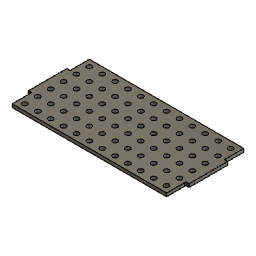
Shelf_Cut1 (Autodesk Fusion 360 design; units mm, degrees)
Autodesk Fusion 360 part; units mm, degrees
sketch "Sketch1" plane through (0, 0, 0) normal (0, 1, 0) x (1, 0, 0)
  line L0 (0, 0) -> (609.6, 0)
  line L1 (609.6, 0) -> (609.6, -304.8)
  line L2 (609.6, -304.8) -> (0, -304.8)
  line L3 (0, -304.8) -> (0, 0)
  line L4 (12.7, -228.6) -> (-12.7, -228.6)
  line L5 (-12.7, -228.6) -> (-12.7, -76.2)
  line L6 (-12.7, -76.2) -> (12.7, -76.2)
  line L7 (12.7, -76.2) -> (12.7, -228.6)
  line L8 (12.7, -228.6) -> (-12.7, -76.2) construction
  line L9 (-12.7, -228.6) -> (12.7, -76.2) construction
  line L10 (622.3, -228.6) -> (596.9, -228.6)
  line L11 (596.9, -228.6) -> (596.9, -76.2)
  line L12 (596.9, -76.2) -> (622.3, -76.2)
  line L13 (622.3, -76.2) -> (622.3, -228.6)
  line L14 (622.3, -228.6) -> (596.9, -76.2) construction
  line L15 (596.9, -228.6) -> (622.3, -76.2) construction
  point P0 (0, -152.4)
  point P1 (609.6, -152.4)
  dimension "d1" = 609.6
  dimension "d2" = 304.8
  dimension "d3" = 25.4
  dimension "d4" = 152.4
  dimension "d5" = 25.4
  dimension "d6" = 152.4
  constraint horizontal L0
  constraint vertical L1
  constraint horizontal L2
  constraint vertical L3
  constraint coincident L0.start L3.end
  constraint horizontal L4
  constraint perpendicular L4 L5
  constraint parallel L4 L6
  constraint parallel L5 L7
  constraint coincident L8 P0
  constraint coincident L9 P0
  constraint midpoint L3 P0
  constraint horizontal L10
  constraint perpendicular L10 L11
  constraint parallel L10 L12
  constraint parallel L11 L13
  constraint coincident L14 P1
  constraint coincident L15 P1
  constraint midpoint L1 P1
  measures "d1" distance of L0.start L0.end
  measures "d2" distance of L0.start L2.end
  measures "d3" distance of L5.end L6.end
  measures "d4" distance of L4.end L5.end
  measures "d5" distance of L11.end L12.end
  measures "d6" distance of L10.end L11.end
extrude "Extrude1" add sketch "Sketch1" along normal blind 12.7 makes body 1 in component "Component"
sketch "Sketch2" plane through (0, 12.7, 0) normal (0, 1, 0) x (-1, 0, 0)
  line L0 (-622.3, 76.2) -> (-609.6, 76.2)
  line L1 (-609.6, 76.2) -> (-609.6, 0)
  line L2 (-609.6, 0) -> (0, 0)
  line L3 (0, 0) -> (0, 76.2)
  line L4 (0, 76.2) -> (12.7, 76.2)
  line L5 (12.7, 76.2) -> (12.7, 228.6)
  line L6 (12.7, 228.6) -> (0, 228.6)
  line L7 (0, 228.6) -> (0, 304.8)
  line L8 (0, 304.8) -> (-609.6, 304.8)
  line L9 (-609.6, 304.8) -> (-609.6, 228.6)
  line L10 (-609.6, 228.6) -> (-622.3, 228.6)
  line L11 (-622.3, 228.6) -> (-622.3, 76.2)
  line L12 (0, 0) -> (-25.4, 0) construction
  line L13 (-25.4, 0) -> (-25.4, 25.4) construction
  circle A0 centre (-25.4, 25.4) radius 9.525
  circle A1 centre (-76.2, 25.4) radius 9.525
  circle A2 centre (-127, 25.4) radius 9.525
  circle A3 centre (-177.8, 25.4) radius 9.525
  circle A4 centre (-228.6, 25.4) radius 9.525
  circle A5 centre (-279.4, 25.4) radius 9.525
  circle A6 centre (-330.2, 25.4) radius 9.525
  circle A7 centre (-381, 25.4) radius 9.525
  circle A8 centre (-431.8, 25.4) radius 9.525
  circle A9 centre (-482.6, 25.4) radius 9.525
  circle A10 centre (-533.4, 25.4) radius 9.525
  circle A11 centre (-584.2, 25.4) radius 9.525
  circle A12 centre (-25.4, 76.2) radius 9.525
  circle A13 centre (-76.2, 76.2) radius 9.525
  circle A14 centre (-127, 76.2) radius 9.525
  circle A15 centre (-177.8, 76.2) radius 9.525
  circle A16 centre (-228.6, 76.2) radius 9.525
  circle A17 centre (-279.4, 76.2) radius 9.525
  circle A18 centre (-330.2, 76.2) radius 9.525
  circle A19 centre (-381, 76.2) radius 9.525
  circle A20 centre (-431.8, 76.2) radius 9.525
  circle A21 centre (-482.6, 76.2) radius 9.525
  circle A22 centre (-533.4, 76.2) radius 9.525
  circle A23 centre (-584.2, 76.2) radius 9.525
  circle A24 centre (-25.4, 127) radius 9.525
  circle A25 centre (-76.2, 127) radius 9.525
  circle A26 centre (-127, 127) radius 9.525
  circle A27 centre (-177.8, 127) radius 9.525
  circle A28 centre (-228.6, 127) radius 9.525
  circle A29 centre (-279.4, 127) radius 9.525
  circle A30 centre (-330.2, 127) radius 9.525
  circle A31 centre (-381, 127) radius 9.525
  circle A32 centre (-431.8, 127) radius 9.525
  circle A33 centre (-482.6, 127) radius 9.525
  circle A34 centre (-533.4, 127) radius 9.525
  circle A35 centre (-584.2, 127) radius 9.525
  circle A36 centre (-25.4, 177.8) radius 9.525
  circle A37 centre (-76.2, 177.8) radius 9.525
  circle A38 centre (-127, 177.8) radius 9.525
  circle A39 centre (-177.8, 177.8) radius 9.525
  circle A40 centre (-228.6, 177.8) radius 9.525
  circle A41 centre (-279.4, 177.8) radius 9.525
  circle A42 centre (-330.2, 177.8) radius 9.525
  circle A43 centre (-381, 177.8) radius 9.525
  circle A44 centre (-431.8, 177.8) radius 9.525
  circle A45 centre (-482.6, 177.8) radius 9.525
  circle A46 centre (-533.4, 177.8) radius 9.525
  circle A47 centre (-584.2, 177.8) radius 9.525
  circle A48 centre (-25.4, 228.6) radius 9.525
  circle A49 centre (-76.2, 228.6) radius 9.525
  circle A50 centre (-127, 228.6) radius 9.525
  circle A51 centre (-177.8, 228.6) radius 9.525
  circle A52 centre (-228.6, 228.6) radius 9.525
  circle A53 centre (-279.4, 228.6) radius 9.525
  circle A54 centre (-330.2, 228.6) radius 9.525
  circle A55 centre (-381, 228.6) radius 9.525
  circle A56 centre (-431.8, 228.6) radius 9.525
  circle A57 centre (-482.6, 228.6) radius 9.525
  circle A58 centre (-533.4, 228.6) radius 9.525
  circle A59 centre (-584.2, 228.6) radius 9.525
  circle A60 centre (-25.4, 279.4) radius 9.525
  circle A61 centre (-76.2, 279.4) radius 9.525
  circle A62 centre (-127, 279.4) radius 9.525
  circle A63 centre (-177.8, 279.4) radius 9.525
  circle A64 centre (-228.6, 279.4) radius 9.525
  circle A65 centre (-279.4, 279.4) radius 9.525
  circle A66 centre (-330.2, 279.4) radius 9.525
  circle A67 centre (-381, 279.4) radius 9.525
  circle A68 centre (-431.8, 279.4) radius 9.525
  circle A69 centre (-482.6, 279.4) radius 9.525
  circle A70 centre (-533.4, 279.4) radius 9.525
  circle A71 centre (-584.2, 279.4) radius 9.525
  dimension "d9" = 25.4
  dimension "d10" = 25.4
  dimension "d11" = 19.05
  dimension "d14" = -558.8
  dimension "d15" = 254
  constraint coincident L2.end L3.start
  constraint perpendicular L3 L12
  constraint perpendicular L12 L13
  constraint coincident L13.end A0.centre
  measures "d9" distance of L2.end L12.end
  measures "d10" distance of L12.end L13.end
  measures "d11" diameter of A0
extrude "Extrude1'" add sketch "Sketch2" along normal blind 12.7 separate body makes body 2 in component "Component'"
ref_plane "WorkPlane1" through (0, 12.7, 228.6) normal (0, 1, 0) x (-1, 0, 0)
sketch "Sketch3" plane through (0, 12.7, 228.6) normal (0, 1, 0) x (-1, 0, 0)
  line L0 (12.7, 0) -> (0, 0) construction
  line L1 (0, 0) -> (0, 76.2) construction
  line L2 (0, 0) -> (2.2451, 2.2451) construction
  circle A0 centre (2.2451, 2.2451) radius 3.175
  dimension "d19" = 3.175
  constraint coincident L0.end L1.start
  constraint coincident L0.end A0
  measures "d19" distance of L0.end L2.end
sweep "Sweep1" cut kept parallel profiles "Sketch3" along 1 edges at (0, 19.05, 228.6) section 1 on bodies 2 bodies 2 in component "Component'"
ref_plane "WorkPlane2" through (0, 12.7, 76.2) normal (0, 1, 0) x (-1, 0, 0)
sketch "Sketch4" plane through (0, 12.7, 76.2) normal (0, 1, 0) x (-1, 0, 0)
  line L0 (0, -76.2) -> (0, 0) construction
  line L1 (0, 0) -> (12.7, 0) construction
  line L2 (0, 0) -> (2.2451, -2.2451) construction
  circle A0 centre (2.2451, -2.2451) radius 3.175
  dimension "d27" = 3.175
  constraint coincident L0.end L1.start
  constraint coincident L0.end A0
  measures "d27" distance of L0.end L2.end
sweep "Sweep2" cut kept parallel profiles "Sketch4" along 1 edges at (0, 19.05, 76.2) section 1 on bodies 2 bodies 2 in component "Component'"
ref_plane "WorkPlane3" through (609.6, 12.7, 76.2) normal (0, 1, 0) x (-1, 0, 0)
sketch "Sketch5" plane through (609.6, 12.7, 76.2) normal (0, 1, 0) x (-1, 0, 0)
  line L0 (-12.7, 0) -> (0, 0) construction
  line L1 (0, 0) -> (0, -76.2) construction
  line L2 (0, 0) -> (-2.2451, -2.2451) construction
  circle A0 centre (-2.2451, -2.2451) radius 3.175
  dimension "d35" = 3.175
  constraint coincident L0.end L1.start
  constraint coincident L0.end A0
  measures "d35" distance of L0.end L2.end
sweep "Sweep3" cut kept parallel profiles "Sketch5" along 1 edges at (609.6, 19.05, 76.2) section 1 on bodies 2 bodies 2 in component "Component'"
ref_plane "WorkPlane4" through (609.6, 12.7, 228.6) normal (0, 1, 0) x (-1, 0, 0)
sketch "Sketch6" plane through (609.6, 12.7, 228.6) normal (0, 1, 0) x (-1, 0, 0)
  line L0 (0, 76.2) -> (0, 0) construction
  line L1 (0, 0) -> (-12.7, 0) construction
  line L2 (0, 0) -> (-2.2451, 2.2451) construction
  circle A0 centre (-2.2451, 2.2451) radius 3.175
  dimension "d43" = 3.175
  constraint coincident L0.end L1.start
  constraint coincident L0.end A0
  measures "d43" distance of L0.end L2.end
sweep "Sweep4" cut kept parallel profiles "Sketch6" along 1 edges at (609.6, 19.05, 228.6) section 1 on bodies 2 bodies 2 in component "Component'"
component "Component" placed x (1, 0, 0) y (0, 1, 0) z (0, 0, 1) at (0, 0, 0)
component "Component'" placed x (1, 0, 0) y (0, 1, 0) z (0, 0, 1) at (0, 0, 0)
equation "d19 = 0.25 in / 2 + 0.00 in"
equation "d27 = 0.25 in / 2 + 0.00 in"
equation "d35 = 0.25 in / 2 + 0.00 in"
equation "d43 = 0.25 in / 2 + 0.00 in"
